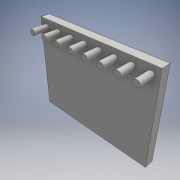
# Autodesk Inventor part: MPU-6050
Saved by Autodesk Inventor 2016 (Build 200138000, 138)
## iProperties
Created: 2015-04-23
Part Number: MPU-6050
Material: Generic
Document SubType Name: Modeling
Designer: StjerneIdioten
Density: 1 g/cm^3
Appearance: Default
Author: StjerneIdioten
Autodesk Inventor part; units mm, degrees
ref_plane "YZ Plane" through (0, 0, 0) normal (1, 0, 0) x (0, 1, 0)
ref_plane "XZ Plane" through (0, 0, 0) normal (0, 1, 0) x (-1, 0, 0)
ref_plane "XY Plane" through (0, 0, 0) normal (0, 0, 1) x (1, 0, 0)
sketch "Sketch4" plane through (0, 0, 0) normal (0, 1, 0) x (-1, 0, 0)
  line L0 (10.125, 7.625) -> (-10.125, 7.625)
  line L1 (-10.125, 7.625) -> (-10.125, -7.625)
  line L2 (-10.125, -7.625) -> (10.125, -7.625)
  line L3 (10.125, -7.625) -> (10.125, 7.625)
  line L4 (10.125, 7.625) -> (-10.125, -7.625) construction
  line L5 (-10.125, 7.625) -> (10.125, -7.625) construction
  point P0 (0, 0)
  dimension "d9" = 20.25
  dimension "d10" = 15.25
  constraints: 12 end point, 2 midpoint, 2 parallel, 1 horizontal, 1 perpendicular
  measures "d9" distance of L2.end L1.end
  measures "d10" distance of L1.end L0.end
extrude "Extrusion2" add sketch "Sketch4" along normal blind 1.5
sketch "Sketch5" plane through (0, 1.5, 0) normal (0, 1, 0) x (1, 0, 0)
  line L0 (-10.125, -7.625) -> (10.125, -7.625) projected
  line L1 (10.125, -7.625) -> (10.125, 7.625) projected
  line L2 (10.125, 7.625) -> (-10.125, 7.625) projected
  line L3 (-10.125, 7.625) -> (-10.125, -7.625) projected
  circle A0 centre (-8.875, -6.375) radius 0.5
  circle A1 centre (-6.335, -6.375) radius 0.5
  circle A2 centre (-3.795, -6.375) radius 0.5
  circle A3 centre (-1.255, -6.375) radius 0.5
  circle A4 centre (1.285, -6.375) radius 0.5
  circle A5 centre (3.825, -6.375) radius 0.5
  circle A6 centre (6.365, -6.375) radius 0.5
  circle A7 centre (8.905, -6.375) radius 0.5
  point P0 (0, 0)
  dimension "d13" = 1
  constraints: 8 centre point
  measures "d13" diameter of A0
extrude "Extrusion3" add sketch "Sketch5" along normal blind 0.5 and the other way blind 4 contours A0 | A1 | A2 | A3 | A4 | A5 | A6 | A7
body "Solid2"
